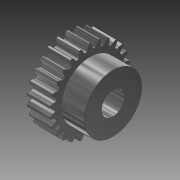
# Autodesk Inventor part: M-0.5 Zb-4mm M-0.7 Zb-5mm mN 21102600
Saved by Autodesk Inventor 2019.3 (Build 233278000, 278)
## iProperties
Category: PARTsolutions
Company: MAEDLER
Created: 2018-08-17
Part Number: M-0.5 Zb-4mm M-0.7 Zb-5mm mN 21102600
Material: Stahl, Guss
Catalog Web Link: www.cadenas.de
Description: M-0.5 Zb-4mm M-0.7 Zb-5mm mN-Spur Gears, Steel, Module 0.5 and 0,7
Vendor: MAEDLER
Document SubType Name: Modeling
Designer: psadmin
Manufacturer: MAEDLER
Mass: 5 g
Surface Area: 7.7022 cm^2
Volume: 0.737711 cm^3
Density: 6.77772 g/cm^3
Appearance: Halbpoliert
PSOL_IDENT_0: {$CADENAS_DATA\23d-libs\maedler\antriebselemente\stirnzahnraeder\stirnzahnraeder_stahl\modul_0.5_und
PSOL_IDENT_1: _0.7\m-0.5_zb-4mm_m-0.7_zb-5mm_mn.prj},237 {VTYP=3D},{NB=M-0.5 Zb-4mm M-0.7 Zb-5mm mN 21102600},{LIN
PSOL_IDENT_2: A=M-0.5 Zb-4mm M-0.7 Zb-5mm mN 21102600},{NN=M-0.5 Zb-4mm M-0.7 Zb-5mm mN},{DATE=27.10.2015 07:21:56
PSOL_IDENT_3: },{GEOMDATE=11.05.2009 09:51:00},{VERSION=},{LINEID=160},{WBVAR=},{WBNUMERIC=}  {NB=M-0.5 Zb-4mm M-0
PSOL_IDENT_4: .7 Zb-5mm mN 21102600},{LINA=M-0.5 Zb-4mm M-0.7 Zb-5mm mN 21102600},{KT=DUMMY},{ARTNR=21102600},{WST=
PSOL_IDENT_5: 11SMnPb30},{M=0.5},{Z=26},{PDF=PDF Katalogseite},{B1=4.0},{DA=14.00},{D=13.00},{NL=4},{ND=10},{B=4},
PSOL_IDENT_6: {MD=4.0},{GEW=5.000}
NN: M-0.5 Zb-4mm M-0.7 Zb-5mm mN
NT: Spur Gears, Steel, Module 0.5 and 0,7
NB: M-0.5 Zb-4mm M-0.7 Zb-5mm mN 21102600
NBSYN: M-0.5 Zb-4mm M-0.7 Zb-5mm mN $ARTNR.
LINA: M-0.5 Zb-4mm M-0.7 Zb-5mm mN 21102600
ARTNR: 21102600
WST: 11SMnPb30
M: 0.5
Z: 26
PDF: PDF Katalogseite
B1: 4
DA: 14
D: 13
NL: 4
ND: 10
B: 4
MD: 4
GEW: 5
SUPPLIER: MAEDLER
ARTICLENO: M-0.5 Zb-4mm M-0.7 Zb-5mm mN 21102600
BOMINFO: M-0.5 Zb-4mm M-0.7 Zb-5mm mN 21102600
CREATOR: CADENAS GmbH
Title: M-0.5 Zb-4mm M-0.7 Zb-5mm mN 21102600
Author: Cadenas PARTsolutions
Comments: Spur Gears, Steel, Module 0.5 and 0,7
Autodesk Inventor part; units mm, degrees
ref_plane "YZ Plane" through (0, 0, 0) normal (1, 0, 0) x (0, 1, 0)
ref_plane "XZ Plane" through (0, 0, 0) normal (0, 1, 0) x (-1, 0, 0)
ref_plane "XY Plane" through (0, 0, 0) normal (0, 0, 1) x (1, 0, 0)
sketch "Skizze_1" plane through (0, 0, 0) normal (1, 0, 0) x (0, 1, 0)
  arc A0 (0.1667, 6.998) -> (-0.1667, 6.998) centre (0, 0) ccw
  line L0 (-0.1667, 6.998) -> (-0.3645, 6.4898)
  line L1 (-0.3645, 6.4898) -> (-0.4828, 5.9805)
  arc A1 (-0.4828, 5.9805) -> (-0.9625, 5.9223) centre (0, 0) ccw
  line L2 (-0.9625, 5.9223) -> (-1.1992, 6.3884)
  line L3 (-1.1992, 6.3884) -> (-1.5129, 6.8346)
  arc A2 (-1.5129, 6.8346) -> (-1.8366, 6.7548) centre (0, 0) ccw
  line L4 (-1.8366, 6.7548) -> (-1.907, 6.214)
  line L5 (-1.907, 6.214) -> (-1.9, 5.6912)
  arc A3 (-1.9, 5.6912) -> (-2.3518, 5.5199) centre (0, 0) ccw
  line L6 (-2.3518, 5.5199) -> (-2.6932, 5.9158)
  line L7 (-2.6932, 5.9158) -> (-3.1046, 6.2739)
  arc A4 (-3.1046, 6.2739) -> (-3.3997, 6.119) centre (0, 0) ccw
  line L8 (-3.3997, 6.119) -> (-3.3387, 5.577)
  line L9 (-3.3387, 5.577) -> (-3.2068, 5.0711)
  arc A5 (-3.2068, 5.0711) -> (-3.6045, 4.7967) centre (0, 0) ccw
  line L10 (-3.6045, 4.7967) -> (-4.0307, 5.0994)
  line L11 (-4.0307, 5.0994) -> (-4.5158, 5.3486)
  arc A6 (-4.5158, 5.3486) -> (-4.7653, 5.1276) centre (0, 0) ccw
  line L12 (-4.7653, 5.1276) -> (-4.5764, 4.6159)
  line L13 (-4.5764, 4.6159) -> (-4.3272, 4.1563)
  arc A7 (-4.3272, 4.1563) -> (-4.6476, 3.7947) centre (0, 0) ccw
  line L14 (-4.6476, 3.7947) -> (-5.1339, 3.9866)
  line L15 (-5.1339, 3.9866) -> (-5.6646, 4.1125)
  arc A8 (-5.6646, 4.1125) -> (-5.8539, 3.8382) centre (0, 0) ccw
  line L16 (-5.8539, 3.8382) -> (-5.548, 3.3866)
  line L17 (-5.548, 3.3866) -> (-5.1962, 3)
  arc A9 (-5.1962, 3) -> (-5.4207, 2.5722) centre (0, 0) ccw
  line L18 (-5.4207, 2.5722) -> (-5.9388, 2.6421)
  line L19 (-5.9388, 2.6421) -> (-6.4842, 2.6374)
  arc A10 (-6.4842, 2.6374) -> (-6.6024, 2.3257) centre (0, 0) ccw
  line L20 (-6.6024, 2.3257) -> (-6.1973, 1.9605)
  line L21 (-6.1973, 1.9605) -> (-5.7631, 1.6693)
  arc A11 (-5.7631, 1.6693) -> (-5.8787, 1.2002) centre (0, 0) ccw
  line L22 (-5.8787, 1.2002) -> (-6.3985, 1.1441)
  line L23 (-6.3985, 1.1441) -> (-6.9269, 1.009)
  arc A12 (-6.9269, 1.009) -> (-6.9671, 0.6781) centre (0, 0) ccw
  line L24 (-6.9671, 0.6781) -> (-6.4864, 0.4204)
  line L25 (-6.4864, 0.4204) -> (-5.9951, 0.2416)
  arc A13 (-5.9951, 0.2416) -> (-5.9951, -0.2416) centre (0, 0) ccw
  line L26 (-5.9951, -0.2416) -> (-6.4864, -0.4204)
  line L27 (-6.4864, -0.4204) -> (-6.9671, -0.6781)
  arc A14 (-6.9671, -0.6781) -> (-6.9269, -1.009) centre (0, 0) ccw
  line L28 (-6.9269, -1.009) -> (-6.3985, -1.1441)
  line L29 (-6.3985, -1.1441) -> (-5.8787, -1.2002)
  arc A15 (-5.8787, -1.2002) -> (-5.7631, -1.6693) centre (0, 0) ccw
  line L30 (-5.7631, -1.6693) -> (-6.1973, -1.9605)
  line L31 (-6.1973, -1.9605) -> (-6.6024, -2.3257)
  arc A16 (-6.6024, -2.3257) -> (-6.4842, -2.6374) centre (0, 0) ccw
  line L32 (-6.4842, -2.6374) -> (-5.9388, -2.6421)
  line L33 (-5.9388, -2.6421) -> (-5.4207, -2.5722)
  arc A17 (-5.4207, -2.5722) -> (-5.1962, -3) centre (0, 0) ccw
  line L34 (-5.1962, -3) -> (-5.548, -3.3866)
  line L35 (-5.548, -3.3866) -> (-5.8539, -3.8382)
  arc A18 (-5.8539, -3.8382) -> (-5.6646, -4.1125) centre (0, 0) ccw
  line L36 (-5.6646, -4.1125) -> (-5.1339, -3.9866)
  line L37 (-5.1339, -3.9866) -> (-4.6476, -3.7947)
  arc A19 (-4.6476, -3.7947) -> (-4.3272, -4.1563) centre (0, 0) ccw
  line L38 (-4.3272, -4.1563) -> (-4.5764, -4.6159)
  line L39 (-4.5764, -4.6159) -> (-4.7653, -5.1276)
  arc A20 (-4.7653, -5.1276) -> (-4.5158, -5.3486) centre (0, 0) ccw
  line L40 (-4.5158, -5.3486) -> (-4.0307, -5.0994)
  line L41 (-4.0307, -5.0994) -> (-3.6045, -4.7967)
  arc A21 (-3.6045, -4.7967) -> (-3.2068, -5.0711) centre (0, 0) ccw
  line L42 (-3.2068, -5.0711) -> (-3.3387, -5.577)
  line L43 (-3.3387, -5.577) -> (-3.3997, -6.119)
  arc A22 (-3.3997, -6.119) -> (-3.1046, -6.2739) centre (0, 0) ccw
  line L44 (-3.1046, -6.2739) -> (-2.6932, -5.9158)
  line L45 (-2.6932, -5.9158) -> (-2.3518, -5.5199)
  arc A23 (-2.3518, -5.5199) -> (-1.9, -5.6912) centre (0, 0) ccw
  line L46 (-1.9, -5.6912) -> (-1.907, -6.214)
  line L47 (-1.907, -6.214) -> (-1.8366, -6.7548)
  arc A24 (-1.8366, -6.7548) -> (-1.5129, -6.8346) centre (0, 0) ccw
  line L48 (-1.5129, -6.8346) -> (-1.1992, -6.3884)
  line L49 (-1.1992, -6.3884) -> (-0.9625, -5.9223)
  arc A25 (-0.9625, -5.9223) -> (-0.4828, -5.9805) centre (0, 0) ccw
  line L50 (-0.4828, -5.9805) -> (-0.3645, -6.4898)
  line L51 (-0.3645, -6.4898) -> (-0.1667, -6.998)
  arc A26 (-0.1667, -6.998) -> (0.1667, -6.998) centre (0, 0) ccw
  line L52 (0.1667, -6.998) -> (0.3645, -6.4898)
  line L53 (0.3645, -6.4898) -> (0.4828, -5.9805)
  arc A27 (0.4828, -5.9805) -> (0.9625, -5.9223) centre (0, 0) ccw
  line L54 (0.9625, -5.9223) -> (1.1992, -6.3884)
  line L55 (1.1992, -6.3884) -> (1.5129, -6.8346)
  arc A28 (1.5129, -6.8346) -> (1.8366, -6.7548) centre (0, 0) ccw
  line L56 (1.8366, -6.7548) -> (1.907, -6.214)
  line L57 (1.907, -6.214) -> (1.9, -5.6912)
  arc A29 (1.9, -5.6912) -> (2.3518, -5.5199) centre (0, 0) ccw
  line L58 (2.3518, -5.5199) -> (2.6932, -5.9158)
  line L59 (2.6932, -5.9158) -> (3.1046, -6.2739)
  arc A30 (3.1046, -6.2739) -> (3.3997, -6.119) centre (0, 0) ccw
  line L60 (3.3997, -6.119) -> (3.3387, -5.577)
  line L61 (3.3387, -5.577) -> (3.2068, -5.0711)
  arc A31 (3.2068, -5.0711) -> (3.6045, -4.7967) centre (0, 0) ccw
  line L62 (3.6045, -4.7967) -> (4.0307, -5.0994)
  line L63 (4.0307, -5.0994) -> (4.5158, -5.3486)
  arc A32 (4.5158, -5.3486) -> (4.7653, -5.1276) centre (0, 0) ccw
  line L64 (4.7653, -5.1276) -> (4.5764, -4.6159)
  line L65 (4.5764, -4.6159) -> (4.3272, -4.1563)
  arc A33 (4.3272, -4.1563) -> (4.6476, -3.7947) centre (0, 0) ccw
  line L66 (4.6476, -3.7947) -> (5.1339, -3.9866)
  line L67 (5.1339, -3.9866) -> (5.6646, -4.1125)
  arc A34 (5.6646, -4.1125) -> (5.8539, -3.8382) centre (0, 0) ccw
  line L68 (5.8539, -3.8382) -> (5.548, -3.3866)
  line L69 (5.548, -3.3866) -> (5.1962, -3)
  arc A35 (5.1962, -3) -> (5.4207, -2.5722) centre (0, 0) ccw
  line L70 (5.4207, -2.5722) -> (5.9388, -2.6421)
  line L71 (5.9388, -2.6421) -> (6.4842, -2.6374)
  arc A36 (6.4842, -2.6374) -> (6.6024, -2.3257) centre (0, 0) ccw
  line L72 (6.6024, -2.3257) -> (6.1973, -1.9605)
  line L73 (6.1973, -1.9605) -> (5.7631, -1.6693)
  arc A37 (5.7631, -1.6693) -> (5.8787, -1.2002) centre (0, 0) ccw
  line L74 (5.8787, -1.2002) -> (6.3985, -1.1441)
  line L75 (6.3985, -1.1441) -> (6.9269, -1.009)
  arc A38 (6.9269, -1.009) -> (6.9671, -0.6781) centre (0, 0) ccw
  line L76 (6.9671, -0.6781) -> (6.4864, -0.4204)
  line L77 (6.4864, -0.4204) -> (5.9951, -0.2416)
  arc A39 (5.9951, -0.2416) -> (5.9951, 0.2416) centre (0, 0) ccw
  line L78 (5.9951, 0.2416) -> (6.4864, 0.4204)
  line L79 (6.4864, 0.4204) -> (6.9671, 0.6781)
  arc A40 (6.9671, 0.6781) -> (6.9269, 1.009) centre (0, 0) ccw
  line L80 (6.9269, 1.009) -> (6.3985, 1.1441)
  line L81 (6.3985, 1.1441) -> (5.8787, 1.2002)
  arc A41 (5.8787, 1.2002) -> (5.7631, 1.6693) centre (0, 0) ccw
  line L82 (5.7631, 1.6693) -> (6.1973, 1.9605)
  line L83 (6.1973, 1.9605) -> (6.6024, 2.3257)
  arc A42 (6.6024, 2.3257) -> (6.4842, 2.6374) centre (0, 0) ccw
  line L84 (6.4842, 2.6374) -> (5.9388, 2.6421)
  line L85 (5.9388, 2.6421) -> (5.4207, 2.5722)
  arc A43 (5.4207, 2.5722) -> (5.1962, 3) centre (0, 0) ccw
  line L86 (5.1962, 3) -> (5.548, 3.3866)
  line L87 (5.548, 3.3866) -> (5.8539, 3.8382)
  arc A44 (5.8539, 3.8382) -> (5.6646, 4.1125) centre (0, 0) ccw
  line L88 (5.6646, 4.1125) -> (5.1339, 3.9866)
  line L89 (5.1339, 3.9866) -> (4.6476, 3.7947)
  arc A45 (4.6476, 3.7947) -> (4.3272, 4.1563) centre (0, 0) ccw
  line L90 (4.3272, 4.1563) -> (4.5764, 4.6159)
  line L91 (4.5764, 4.6159) -> (4.7653, 5.1276)
  arc A46 (4.7653, 5.1276) -> (4.5158, 5.3486) centre (0, 0) ccw
  line L92 (4.5158, 5.3486) -> (4.0307, 5.0994)
  line L93 (4.0307, 5.0994) -> (3.6045, 4.7967)
  arc A47 (3.6045, 4.7967) -> (3.2068, 5.0711) centre (0, 0) ccw
  line L94 (3.2068, 5.0711) -> (3.3387, 5.577)
  line L95 (3.3387, 5.577) -> (3.3997, 6.119)
  arc A48 (3.3997, 6.119) -> (3.1046, 6.2739) centre (0, 0) ccw
  line L96 (3.1046, 6.2739) -> (2.6932, 5.9158)
  line L97 (2.6932, 5.9158) -> (2.3518, 5.5199)
  arc A49 (2.3518, 5.5199) -> (1.9, 5.6912) centre (0, 0) ccw
  line L98 (1.9, 5.6912) -> (1.907, 6.214)
  line L99 (1.907, 6.214) -> (1.8366, 6.7548)
  arc A50 (1.8366, 6.7548) -> (1.5129, 6.8346) centre (0, 0) ccw
  line L100 (1.5129, 6.8346) -> (1.1992, 6.3884)
  line L101 (1.1992, 6.3884) -> (0.9625, 5.9223)
  arc A51 (0.9625, 5.9223) -> (0.4828, 5.9805) centre (0, 0) ccw
  line L102 (0.4828, 5.9805) -> (0.3645, 6.4898)
  line L103 (0.3645, 6.4898) -> (0.1667, 6.998)
  constraints: 208 end point, 104 point on circle, 52 centre point
extrude "Extrusion1" add sketch "Skizze_1" along normal mid plane 4
sketch "Skizze_2" plane through (0, 0, 0) normal (0, 0, 1) x (1, 0, 0)
  line L0 (6, 0) -> (2, 0)
  line L1 (2, 0) -> (2, 5)
  line L2 (2, 5) -> (6, 5)
  line L3 (6, 5) -> (6, 0)
  line L4 (6, 0) -> (2, 0)
  constraints: 10 end point
revolve "Revolution1" add sketch "Skizze_2" angle 360 about axis through (6, 0, 0) along (1, 0, 0)
sketch "Skizze_3" plane through (6, 0, 0) normal (1, 0, 0) x (0, 1, 0)
  circle A0 centre (0, 0) radius 2
  constraints: 1 centre point
extrude "Extrusion2" cut sketch "Skizze_3" along normal mid plane 16
body "Solid1"
